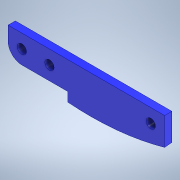
# Autodesk Inventor part: Upper blade
Saved by Autodesk Inventor 2020.3 (Build 243373000, 373)
## iProperties
Created: 2021-06-11
Part Number: Upper blade
Material: Generic
Document SubType Name: Modeling
Designer: User
Density: 1 g/cm^3
Appearance: Blue - Wall Paint - Glossy
Author: User
Autodesk Inventor part; units mm, degrees
ref_plane "YZ Plane" through (0, 0, 0) normal (1, 0, 0) x (0, 1, 0)
ref_plane "XZ Plane" through (0, 0, 0) normal (0, 1, 0) x (-1, 0, 0)
ref_plane "XY Plane" through (0, 0, 0) normal (0, 0, 1) x (1, 0, 0)
sketch "Sketch1" plane through (0, 0, 0) normal (0, 0, 1) x (1, 0, 0)
  line L0 (0, -30) -> (0, 0)
  line L1 (0, 0) -> (-170, 0)
  line L2 (-170, 0) -> (-170, -15)
  line L3 (-155, -30) -> (-105, -30)
  line L4 (-105, -30) -> (-105, -40)
  arc A0 (-105, -40) -> (0, -30) centre (-80.4998, 258.9979) ccw
  arc A1 (-170, -15) -> (-155, -30) centre (-155, -15) ccw
  circle A2 centre (-155, -15) radius 5
  circle A3 centre (-125, -15) radius 5
  circle A4 centre (-15, -15) radius 5
  point P0 (-170, -30)
  dimension "d0" = 170
  dimension "d1" = 30
  dimension "d2" = 30
  dimension "d3" = 65
  dimension "d4" = 10
  dimension "d6" = 300
  dimension "d7" = 15
  dimension "d8" = 10
  dimension "d9" = 10
  dimension "d10" = 10
  dimension "d11" = 15
  dimension "d12" = 30
  dimension "d13" = 15
  dimension "d14" = 15
  constraints: 10 end point, 5 centre point, 4 perpendicular, 4 point on circle, 2 horizontal alignment, 2 point on line, 2 tangent, 1 vertical
  measures "d0" distance of L0.end L1.end
  measures "d1" distance of L0.start L0.end
  measures "d2" distance of L1.end point (-170, -30)
  measures "d3" distance of point (-170, -30) L3.end
  measures "d4" distance of L3.end L4.end
  measures "d6" radius of A0
  measures "d7" radius of A1
  measures "d8" diameter of A2
  measures "d9" diameter of A3
  measures "d10" diameter of A4
  measures "d11" distance of L2.end A2.centre
  measures "d12" distance of A3.centre A1.centre
  measures "d13" distance from line of L0 A4.centre
  measures "d14" distance from line of L1 A4.centre
extrude "Extrusion1" add sketch "Sketch1" along normal blind 7.9375
chamfer "Chamfer1" distance 7.9375 angle 5 1 edges at (-52.0571, -39.6507, 0) measured on face at (-48.5408, -39.295, 5.2917)
body "Solid1"
